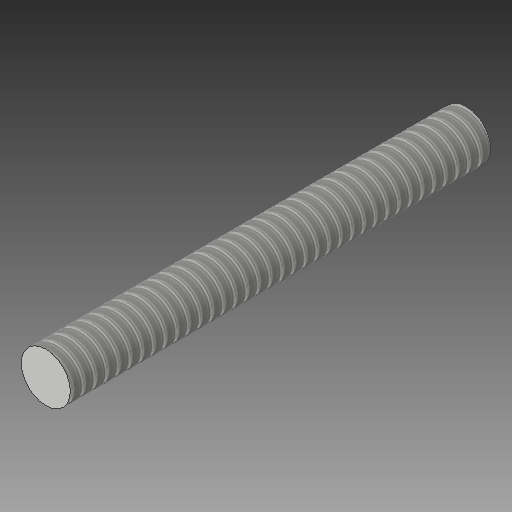
# Autodesk Inventor part: RollerThing2
Saved by Autodesk Inventor 2018 (Build 220112000, 112)
## iProperties
Created: 2020-01-24
Part Number: RollerThing2
Material: Generic
Document SubType Name: Modeling
Designer: 22perngrac
Density: 1 g/cm^3
Appearance: Default
Mass: 0.591233 g
Surface Area: 5.63079 cm^2
Volume: 0.591233 cm^3
Author: 22perngrac
Autodesk Inventor part; units mm, degrees
ref_plane "YZ Plane" through (0, 0, 0) normal (1, 0, 0) x (0, 1, 0)
ref_plane "XZ Plane" through (0, 0, 0) normal (0, 1, 0) x (-1, 0, 0)
sketch "Sketch1" plane through (0, 0, 0) normal (0, 0, 1) x (1, 0, 0)
  circle A0 centre (0, 0) radius 2.2225
  dimension "d0" = 4.445
  constraints: 1 centre point, 1 coincident
  measures "d0" diameter of A0
extrude "Extrusion1" add sketch "Sketch1" along normal blind 38.1
thread "Thread1" size "10-24 UNC" class "2A" standard "ANSI Unified Screw Threads" full length
ref_plane "Work Plane1" through (0, 0, 19.05) normal (0, 0, 1) x (1, 0, 0)
body "Solid1"
